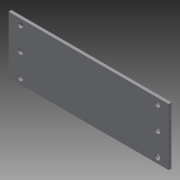
# Autodesk Inventor part: base and top plate real
Saved by Autodesk Inventor 2015 (Build 190159000, 159)
## iProperties
Created: 2015-01-20
Part Number: base and top plate real
Material: Generic
Document SubType Name: Modeling
Designer: mastkee16
Density: 1 g/cm^3
Appearance: Default
Author: mastkee16
Autodesk Inventor part; units mm, degrees
ref_plane "YZ Plane" through (0, 0, 0) normal (1, 0, 0) x (0, 1, 0)
ref_plane "XZ Plane" through (0, 0, 0) normal (0, 1, 0) x (-1, 0, 0)
ref_plane "XY Plane" through (0, 0, 0) normal (0, 0, 1) x (1, 0, 0)
sketch "Sketch1" plane through (0, 0, 0) normal (0, 0, 1) x (1, 0, 0)
  line L0 (-0.2558, -58.1023) -> (177.5442, -58.1023)
  line L1 (177.5442, -58.1023) -> (177.5442, 5.3977)
  line L2 (177.5442, 5.3977) -> (-0.2558, 5.3977)
  line L3 (-0.2558, 5.3977) -> (-0.2558, -58.1023)
  point P0 (0, 0)
  dimension "d0" = 177.8
  dimension "d1" = 63.5
  constraints: 8 end point, 2 parallel, 1 horizontal, 1 perpendicular
  measures "d0" distance of L2.end L1.end
  measures "d1" distance of L2.end L0.start
extrude "Extrusion1" add sketch "Sketch1" along normal blind 3.175
sketch "Sketch3" plane through (0, 0, 3.175) normal (0, 0, 1) x (1, 0, 0)
  line L0 (-0.2558, 5.3977) -> (-0.2558, -58.1023) projected
  line L1 (177.5442, 5.3977) -> (-0.2558, 5.3977) projected
  line L2 (-0.2558, -58.1023) -> (177.5442, -58.1023) projected
  line L3 (177.5442, -58.1023) -> (177.5442, 5.3977) projected
  point P0 (0, 0)
  point P1 (12.4442, -0.9523)
  point P2 (12.4442, -26.3523)
  point P3 (12.4442, -51.7523)
  point P4 (164.8442, -0.9523)
  point P5 (164.8442, -26.3523)
  point P6 (164.8442, -51.7523)
  dimension "d22" = 25.4
  dimension "d23" = 25.4
  dimension "d26" = 12.7
  dimension "d27" = 12.7
  dimension "d28" = 12.7
  dimension "d29" = 6.35
  dimension "d30" = 6.35
  dimension "d33" = 6.35
  dimension "d34" = 25.4
  dimension "d35" = 25.4
  dimension "d36" = 12.7
  measures "d22" distance of point (12.444, -26.352) point (12.444, -0.952)
  measures "d23" distance of point (12.444, -26.352) point (12.444, -51.752)
  measures "d26" distance from line of L0 point (12.444, -0.952)
  measures "d27" distance from line of L0 point (12.444, -26.352)
  measures "d28" distance from line of L0 point (12.444, -51.752)
  measures "d29" distance from line of L1 point (12.444, -0.952)
  measures "d30" distance from line of L2 point (12.444, -51.752)
  measures "d33" distance from line of L1 point (164.844, -0.952)
  measures "d34" distance of point (164.844, -26.352) point (164.844, -0.952)
  measures "d35" distance of point (164.844, -26.352) point (164.844, -51.752)
  measures "d36" distance from line of L3 point (164.844, -0.952)
hole "Hole2" at (12.4442, -0.9523, 3.175) at (12.4442, -26.3523, 3.175) at (12.4442, -51.7523, 3.175) at (164.8442, -0.9523, 3.175) at (164.8442, -26.3523, 3.175) at (164.8442, -51.7523, 3.175) direction (0, 0, -1) diameter 6.35 end through all
body "Solid1"
